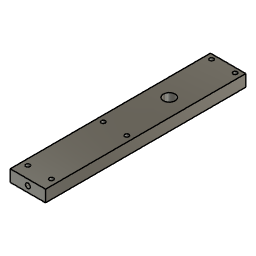
mount_rain (Autodesk Fusion 360 design; units mm, degrees)
Autodesk Fusion 360 part; units mm, degrees
sketch "Sketch1" plane through (0, 0, 0) normal (0, 0, 1) x (1, 0, 0)
  line L0 (15, 85) -> (-15, 85)
  line L1 (-15, 85) -> (-15, -85)
  line L2 (-15, -85) -> (15, -85)
  line L3 (15, -85) -> (15, 85)
  line L4 (15, 85) -> (-15, -85) construction
  line L5 (-15, 85) -> (15, -85) construction
  circle A0 centre (-10, 81) radius 1.75
  circle A1 centre (10, 81) radius 1.75
  circle A2 centre (-10, -11) radius 1.75
  circle A3 centre (10, -11) radius 1.75
  circle A4 centre (-10, -75) radius 1.75
  circle A5 centre (10, -75) radius 1.75
  circle A6 centre (0, 35) radius 5
  dimension "d1" = 30
  dimension "d2" = 170
  dimension "d5" = 4
  dimension "d6" = 4
  dimension "d7" = 10
  dimension "d8" = 10
  dimension "d11" = 10
  dimension "d12" = 10
  dimension "d13" = 92
  dimension "d14" = 92
  dimension "d15" = 3.5
  dimension "d17" = 10
  dimension "d18" = 10
  dimension "d19" = 10
  dimension "d20" = 10
  dimension "d26" = 10
  dimension "d27" = 46
  constraint horizontal L0
  constraint perpendicular L0 L1
  constraint parallel L0 L2
  constraint parallel L1 L3
  constraint coincident L4 origin
  constraint coincident L5 origin
  constraint equal A0 A1
  constraint equal A1 A3
  constraint equal A2 A3
  constraint equal A2 A4
  constraint equal A4 A5
  constraint vertical origin A6.centre
  measures "d1" distance of L1.end L2.end
  measures "d2" distance of L0.end L1.end
  measures "d5" distance of L0 A1.centre
  measures "d6" distance of L0 A0.centre
  measures "d7" horizontal distance of origin A0.centre
  measures "d8" horizontal distance of origin A1.centre
  measures "d11" horizontal distance of origin A3.centre
  measures "d12" horizontal distance of origin A2.centre
  measures "d13" distance of A1.centre A3.centre
  measures "d14" distance of A0.centre A2.centre
  measures "d15" diameter of A4
  measures "d17" horizontal distance of origin A4.centre
  measures "d18" horizontal distance of origin A5.centre
  measures "d19" distance of L2 A4.centre
  measures "d20" distance of L2 A5.centre
  measures "d26" diameter of A6
  measures "d27" vertical distance of A3.centre A6.centre
extrude "Extrude1" add sketch "Sketch1" along normal blind 10
sketch "Sketch2" plane through (0, -85, 0) normal (0, -1, 0) x (1, 0, 0)
  line L0 (-15, 0) -> (15, 0)
  line L1 (15, 0) -> (15, 10)
  line L2 (15, 10) -> (-15, 10)
  line L3 (-15, 10) -> (-15, 0)
  circle A0 centre (0, 5) radius 2.05
  point P0 (15, 5)
  dimension "d23" = 4.1
  constraint vertical origin A0.centre
  constraint midpoint L1 P0
  constraint horizontal A0.centre P0
  measures "d23" diameter of A0
extrude "Extrude2" cut sketch "Sketch2" against normal blind 8 contours A0
sketch "Sketch3" plane through (0, 0, 0) normal (0, 0, -1) x (1, 0, 0)
  circle A0 centre (10, -81) radius 1.75
  circle A1 centre (10, 11) radius 1.75
  circle A2 centre (-10, 11) radius 1.75
  circle A3 centre (-10, 75) radius 1.75
  circle A4 centre (-10, -81) radius 1.75
  circle A5 centre (10, 75) radius 1.75
  circle A6 centre (0, -35) radius 5
  line L0 (15, -85) -> (15, 85)
  line L1 (15, 85) -> (-15, 85)
  line L2 (-15, 85) -> (-15, -85)
  line L3 (-15, -85) -> (15, -85)
  line L4 (0, -35) -> (0, 75)
  dimension "d28" = 10
  constraint parallel L0 L4
  constraint coincident A6.centre L4.start
  measures "d28" distance of L1 L4.end
pipe "Pipe1" cut diameter 5 path "Sketch3" along L4
fillet "Fillet1" radius 2.5 1 edges at (0, -75, 2.5)
